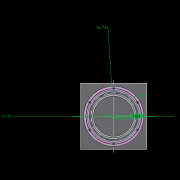
# Autodesk Inventor part: Top_revolOuterBearing_TBS
Saved by Autodesk Inventor 2022.2 (Build 262287010, 287A)
## iProperties
Created: 2022-05-21
Part Number: Top_revolOuterBearing_TBS
Material: Generic
Document SubType Name: Modeling
Designer: Árni Þór Þorgeirsson
Density: 1 g/cm^3
Appearance: Default
Author: Árni Þór Þorgeirsson
Autodesk Inventor part; units mm, degrees
ref_plane "YZ Plane" through (0, 0, 0) normal (1, 0, 0) x (0, 1, 0)
ref_plane "XZ Plane" through (0, 0, 0) normal (0, 1, 0) x (-1, 0, 0)
sketch "Sketch7" plane through (0, 0, 0) normal (0, 1, 0) x (-1, 0, 0)
  line L0 (0, 0) -> (0, 61.9844)
  line L1 (0, 0) -> (-59.2469, 0) construction
  line L2 (0, 61.9844) -> (-59.2469, 0) construction
  line L3 (0, 61.9844) -> (-64.8494, 0) construction
  line L4 (0, 61.9844) -> (-58.9939, -5.5968) construction
  line L5 (0, 0) -> (0, -61.9844)
  line L6 (0, -61.9844) -> (-59.2469, 0) construction
  line L7 (0, -61.9844) -> (-64.8494, 0) construction
  line L8 (0, -61.9844) -> (-58.9939, 5.5968) construction
  line L9 (-58.9939, 5.5968) -> (-64.8494, 0) construction
  line L10 (-54.1083, 0) -> (-62.8579, -8.363) construction
  line L11 (-54.1083, 0) -> (-38.773, -14.6578) construction
  line L12 (0, -94.3812) -> (0, 132.3969) projected
  line L13 (-75, -5.9919) -> (-75, 6.008)
  line L14 (105, 0) -> (-105, 0) projected
  line L15 (-62.0481, 2.6775) -> (-56.4456, -2.6775) construction
  line L16 (-56.4456, 2.6775) -> (-62.0481, -2.6775) construction
  line L17 (-26.151, -15.9303) -> (-40.3783, -15.9303) construction
  line L18 (-40.3783, -15.9303) -> (-40.3783, -12.7539) construction
  line L19 (-40.3783, -12.7539) -> (-26.151, -12.7539) construction
  line L20 (-26.151, -12.7539) -> (-26.151, -15.9303) construction
  point P0 (-75, 0)
  dimension "Roller_Side_difference" = -0.0002
  dimension "d90" = 61.9844
  dimension "d201" = 75
  dimension "d343" = 92.587
  dimension "d344" = 92.588
  dimension "d367" = 8.1
  constraints: 28 end point, 9 point on line, 3 midpoint, 3 vertical, 2 horizontal, 2 parallel, 2 perpendicular, 1 collinear, 1 symmetric about line, 2 other
  measures "d90" distance of L0.start L0.end
  measures "d201" distance between parallel lines of L5 L13
  measures "d343" angle of L10 L8
  measures "d344" angle of L7 L10
  measures "d367" distance of L3.end L8.end
sketch "Sketch1" plane through (0, 0, 0) normal (0, 0, 1) x (1, 0, 0)
  circle A0 centre (0, 0) radius 59.2469 construction
  line L0 (0, 0) -> (59.2469, 0)
  line L1 (0, 0) -> (59.2469, 4.025)
  line L2 (59.2469, 0) -> (59.2469, 4.025)
  circle A1 centre (0, 0) radius 75
  dimension "d56" = 59.2469
  dimension "d57" = 4.025
  dimension "d400" = 75
  dimension "d495" = 2.5
  dimension "d496" = 8
  dimension "d531" = 5.5
  dimension "d532" = 5.5
  dimension "d533" = 5.5
  dimension "d537" = 24.5
  dimension "d538" = 3
  dimension "d543" = 5.5
  dimension "d549" = 3
  dimension "d550" = 3
  dimension "d567" = 5.5
  dimension "d568" = 5.5
  constraints: 1 other
sketch "Roller1" plane through (0, 0, 0) normal (0, 1, 0) x (-1, 0, 0)
  line L0 (0, 61.9844) -> (-58.9939, -5.5968) construction
  line L1 (0, 61.9844) -> (-64.8494, 0) construction
  line L2 (-54.1083, 0) -> (-38.773, -14.6578) construction
  line L3 (0, -61.9844) -> (-64.8494, 0) construction
  line L4 (-54.0606, 0.0927) -> (-58.9462, -5.5041)
  line L5 (-58.9462, -5.5041) -> (-64.7589, 0.0519)
  line L6 (-64.7589, 0.0519) -> (-59.3884, 5.1851)
  line L7 (-59.3884, 5.1851) -> (-54.0606, 0.0927)
  line L8 (-56.0019, 1.9482) -> (-61.1299, -3.4168)
  line L9 (-61.8526, -2.7261) -> (-56.7246, 2.639)
  point P0 (0, 0)
  dimension "d345" = 0.025
  dimension "d346" = 0.025
  dimension "d347" = 0.1
  dimension "d348" = 0.1
  dimension "d349" = 272.588
  dimension "d350" = 272.587
  dimension "d617" = 0.9997
  constraints: 12 end point, 4 parallel, 3 point on line, 1 midpoint, 1 perpendicular
  measures "d345" distance between parallel lines of L0 L4
  measures "d346" distance between parallel lines of L1 L6
  measures "d347" distance between parallel lines of L3 L5
  measures "d348" distance between parallel lines of L2 L7
  measures "d617" distance between parallel lines of L9 L8
sketch "Roller2" plane through (0, 0, 0) normal (0, 1, 0) x (-1, 0, 0)
  line L0 (0, -61.9844) -> (-58.9939, 5.5968) construction
  line L1 (-54.1083, 0) -> (-62.8579, -8.363) construction
  line L2 (0, -61.9844) -> (-64.8494, 0) construction
  line L3 (0, 61.9844) -> (-64.8494, 0) construction
  line L4 (-58.9462, 5.5041) -> (-54.1923, 0.0581)
  line L5 (-54.1923, 0.0581) -> (-59.5331, -5.0468)
  line L6 (-59.5331, -5.0468) -> (-64.7589, -0.0519)
  line L7 (-64.7589, -0.0519) -> (-58.9462, 5.5041)
  line L8 (-61.8526, 2.7261) -> (-56.8627, -2.4944)
  line L9 (-61.1297, 3.417) -> (-56.1399, -1.8034)
  point P0 (0, 0)
  dimension "d351" = 0.025
  dimension "d352" = 0.025
  dimension "d354" = 0.1
  dimension "d355" = 92.587
  dimension "d356" = 92.588
  dimension "d370" = 0.1
  dimension "d371" = 1
  constraints: 12 end point, 5 parallel, 3 point on line, 1 midpoint, 1 perpendicular
  measures "d351" distance between parallel lines of L0 L4
  measures "d352" distance between parallel lines of L2 L6
  measures "d354" distance between parallel lines of L1 L5
  measures "d355" angle of L5 L4
  measures "d356" angle of L6 L5
  measures "d370" distance from line of L3 L8.start
  measures "d371" distance between parallel lines of L9 L8
sketch "Sketch22" plane through (0, 0, 0) normal (0, 1, 0) x (-1, 0, 0)
  line L0 (-31.756, 8.0215) -> (-17.5287, 8.0215) construction
  line L1 (-17.5287, 8.0215) -> (-17.5287, 4.8451) construction
  line L2 (-17.5287, 4.8451) -> (-31.756, 4.8451) construction
  line L3 (-31.756, 4.8451) -> (-31.756, 8.0215) construction
  point P0 (0, 0)
  dimension "Roller_Side_difference" = -0.0002
  constraints: 2 other
sketch "Sketch2" plane through (0, 0, 0) normal (0, 1, 0) x (-1, 0, 0)
  line L0 (0, 0) -> (0, 59.2469) construction
  line L1 (0, 0) -> (-59.2469, 0) projected
  line L2 (0, 0) -> (0, -59.2469)
  line L3 (0, -59.2469) -> (-59.2469, 0) construction
  line L4 (0, 59.2469) -> (-59.2469, 0) construction
  line L5 (-50.488, 53.5552) -> (0, 59.2469) construction
  line L6 (-29.7354, 7.189) -> (0, 59.2469) construction
  line L7 (-29.7354, 7.189) -> (0, -59.2469) construction
  line L8 (-48.8381, -26.254) -> (0, -59.2469) construction
  point P0 (-40.4258, 18.8211)
  constraints: 16 end point, 3 point on line, 1 perpendicular, 1 symmetric about line, 1 vertical
sketch "Sketch23" plane through (0, 0, 0) normal (0, 1, 0) x (-1, 0, 0)
  line L0 (0, -61.9844) -> (-58.9939, 5.5968) construction
  line L1 (0, -61.9844) -> (-64.8494, 0) construction
  line L2 (0, 61.9844) -> (-58.9939, -5.5968) construction
  line L3 (-58.9939, 5.5968) -> (-64.8494, 0) construction
  line L4 (0, 61.9844) -> (-64.8494, 0) construction
  line L5 (-58.9939, 5.5968) -> (-58.9939, -5.5968) construction
  line L6 (105, 0) -> (-105, 0) projected
  line L7 (-57.5518, 4.0968) -> (-54.033, 0.0658)
  line L8 (-54.033, -0.0658) -> (-57.5518, -4.0968)
  line L9 (-60.708, 4.0968) -> (-64.9185, 0.0723)
  line L10 (-64.9185, -0.0723) -> (-60.708, -4.0968)
  arc A0 (-64.9185, 0.0723) -> (-64.9185, -0.0723) centre (-64.8494, 0) ccw
  arc A1 (-54.033, -0.0658) -> (-54.033, 0.0658) centre (-54.1083, 0) ccw
  line L11 (-57.5518, 4.0968) -> (-57.5518, 5.5968)
  line L12 (-57.5518, 5.5968) -> (-50, 5.5968)
  line L13 (-50, 5.5968) -> (-50, -5.5968)
  line L14 (-50, -5.5968) -> (-57.5518, -5.5968)
  line L15 (-57.5518, -5.5968) -> (-57.5518, -4.0968)
  line L16 (-60.708, 4.0968) -> (-60.708, 5.5968)
  line L17 (-60.708, 5.5968) -> (-75, 5.5968)
  line L18 (-75, 5.5968) -> (-75, -5.5968)
  line L19 (-60.708, -4.0968) -> (-60.708, -5.5968)
  line L20 (-60.708, -5.5968) -> (-75, -5.5968)
  line L21 (-58.9939, 5.5968) -> (-58.9939, 5.5968)
  line L22 (-58.9939, -5.5968) -> (-58.9939, -5.5968)
  line L23 (0, -94.3812) -> (0, 132.3969) projected
  line L24 (-64.9941, 0) -> (-75, 0)
  point P0 (0, 0)
  point P1 (-53.9756, 0)
  point P2 (-64.9494, 0)
  point P3 (-75, 0)
  dimension "d378" = 90
  dimension "d379" = 0.1
  dimension "d380" = 0.1
  dimension "d381" = 0.1
  dimension "d382" = 0.1
  dimension "d383" = 0.1
  dimension "d384" = 11.1935
  dimension "d385" = 0
  dimension "d386" = 0
  dimension "d391" = 50
  dimension "d392" = 75
  dimension "d393" = 1.5
  dimension "d394" = 1.5
  dimension "d395" = 1.5
  dimension "d396" = 1.5
  constraints: 36 end point, 10 point on line, 9 vertical, 4 horizontal, 4 parallel, 4 point on circle, 4 tangent, 2 centre point, 1 equal radius, 1 midpoint
  measures "d378" angle of L6 L5
  measures "d379" radius of A0
  measures "d380" distance between parallel lines of L9 L4
  measures "d381" distance between parallel lines of L10 L1
  measures "d382" distance between parallel lines of L0 L7
  measures "d383" distance between parallel lines of L2 L8
  measures "d384" distance of L0.end L2.end
  measures "d385" distance of L2.end L22.end
  measures "d386" distance of L0.end L21.end
  measures "d391" distance between parallel lines of L23 L13
  measures "d392" distance between parallel lines of L18 L23
  measures "d393" distance of L9.start L16.end
  measures "d394" distance of L7.start L11.end
  measures "d395" distance of L14.end L8.end
  measures "d396" distance of L10.end L19.end
revolve "RevRoller1" [suppressed]
fillet "Fillet1" [suppressed]
sketch "Sketch40" plane through (0, 0, -5.231) normal (0, 0, -1) x (-1, 0, 0)
  circle A0 centre (53.5, 0) radius 2.75 projected
  circle A1 centre (0, 0) radius 53.5 projected
  point P0 (53.4293, 2.7491)
  point P1 (53.4293, -2.7491)
  dimension "d585" = 8
  dimension "d587" = 1.75
  dimension "d589" = 3
  dimension "d592" = 2
  dimension "d593" = 12
  dimension "d594" = 12
  dimension "d611" = 360
  constraints: 18 point on circle, 10 centre point, 8 end point, 2 midpoint, 1 horizontal alignment, 1 vertical, 29 other
  measures "d589" diameter of A1
pattern_circular "Circular Pattern13" [suppressed]
feature "Move Body7" [suppressed]
revolve "Revolution13" [suppressed]
fillet "Fillet3" [suppressed]
pattern_circular "Circular Pattern14" [suppressed]
feature "Move Body6" [suppressed]
revolve "Revolution14" add sketch "Sketch23" angle 360 about axis through (0, 0, -10) along (0, 0, 1) contours L13 L14 L15 L8 A1 L6 | L6 A1 L7 L11 L12 L13
revolve "OuterRim_Top2" add sketch "Sketch23" angle 360 about axis through (0, 0, -10) along (0, 0, 1) contours L6 A0 L10 L19 L20 L18
revolve "OuterRim_Bottom2" [suppressed]
ref_plane "Work Plane7" through (0, 0, 100) normal (0, 0, 1) x (1, 0, 0)
sketch "Sketch47" plane through (0, 0, 100) normal (0, 0, 1) x (1, 0, 0)
  circle A0 centre (0, 0) radius 75 construction
  circle A1 centre (0, 0) radius 60.708 construction
  circle A2 centre (0, 0) radius 57.5518 construction
  circle A3 centre (0, 0) radius 50 construction
  circle A4 centre (0, 0) radius 69
  point P0 (0, 69)
  dimension "d620" = 69
  constraints: 1 coincident, 1 vertical alignment, 2 other
sketch "Sketch48" plane through (0, 0, 5.5968) normal (0, 0, 1) x (1, 0, 0)
  circle A0 centre (0, 69) radius 2.75
  circle A1 centre (0, 69) radius 1.5
  circle A2 centre (0, 0) radius 69 construction
  dimension "d621" = 3
  dimension "d622" = 5.5
  constraints: 2 centre point, 2 coincident, 1 vertical alignment
  measures "d621" diameter of A1
  measures "d622" diameter of A0
extrude "Extrusion39" [suppressed]
extrude "Extrusion40" [suppressed]
pattern_circular "Circular Pattern28" [suppressed]
sketch "Sketch49" plane through (0, 0, -5.5968) normal (0, 0, -1) x (-1, 0, 0)
  circle A0 centre (0, 0) radius 69 construction
  circle A1 centre (0, 69) radius 1.5
  line L0 (2.75, 67.4123) -> (0, 65.8246)
  line L1 (0, 65.8246) -> (-2.75, 67.4123)
  line L2 (-2.75, 67.4123) -> (-2.75, 70.5877)
  line L3 (-2.75, 70.5877) -> (0, 72.1754)
  line L4 (0, 72.1754) -> (2.75, 70.5877)
  line L5 (2.75, 70.5877) -> (2.75, 67.4123)
  dimension "d630" = 5.5
  dimension "d631" = 3
  constraints: 12 end point, 2 coincident, 1 centre point, 1 vertical alignment, 13 other
  measures "d630" distance between parallel lines of L5 L2
  measures "d631" diameter of A1
extrude "Extrusion41" cut sketch "Sketch49" against normal blind 5.5968 contours A1
extrude "Extrusion42" cut sketch "Sketch49" against normal blind 2.5935
pattern_circular "Circular Pattern29" count 6 over 360 about axis through (0, 0, -4.8468) along (0, 0, 1) of "Extrusion41", "Extrusion42"
equation "\"Roller_Side_difference\" = -0.000942deg"
equation "\"Cycloid_Top_Plate_Fasner_Inner\" = 61.25"
equation "\"Cycloid_Top_Plate_Fasner_Outer\" = 85.75"
equation "\"Roller_Hole_Radius\" = 1"
equation "\"Distance_To_Bearing\" = 85.74529"
equation "\"d514\" = 0.2"
body "Solid1"
body "Solid5"
